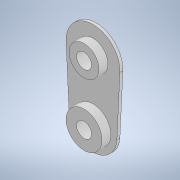
# Autodesk Inventor part: ヘッケン抑え
Saved by Autodesk Inventor 2022.2 (Build 262287030, 287C)
## iProperties
Created: 2022-01-09
Part Number: ヘッケン抑え
Material: Generic
Document SubType Name: Modeling
Designer: acps
Density: 1 g/cm^3
Appearance: Default
Author: acps
Autodesk Inventor part; units mm, degrees
ref_plane "YZ Plane" through (0, 0, 0) normal (1, 0, 0) x (0, 1, 0)
ref_plane "XZ Plane" through (0, 0, 0) normal (0, 1, 0) x (-1, 0, 0)
ref_plane "XY Plane" through (0, 0, 0) normal (0, 0, 1) x (1, 0, 0)
sketch "Sketch1" plane through (0, 0, 0) normal (0, 0, 1) x (1, 0, 0)
  circle A0 centre (0, 0) radius 2.5
  circle A1 centre (0, 0) radius 4.5
  circle A2 centre (0, -10) radius 1.25
  circle A3 centre (0, -10) radius 3
  circle A4 centre (0, -10) radius 4
  circle A5 centre (0, 0) radius 1.25
  line L0 (-4.4944, -0.225) -> (-3.995, -10.2)
  line L1 (4.4944, -0.225) -> (3.995, -10.2)
  line L2 (0, 0) -> (0, -19.0302) construction
  point P0 (66.1895, -52.0583)
  point P1 (148.6808, -39.1685)
  point P2 (99.1548, -7.9801)
  point P3 (101.772, -8.3287)
  point P4 (96.5376, -8.3287)
  dimension "d8" = 9
  dimension "d13" = 5
  dimension "d25" = 2.5
  dimension "d26" = 6
  dimension "d27" = 8
  dimension "d28" = 2.5
  dimension "d29" = 10
  constraints: 7 coincident, 6 centre point, 6 end point, 4 point on circle, 4 tangent, 1 point on line, 1 vertical
  measures "d8" diameter of A1
  measures "d13" diameter of A0
  measures "d25" diameter of A2
  measures "d26" diameter of A3
  measures "d27" diameter of A4
  measures "d28" diameter of A5
  measures "d29" distance of A2.centre point (0, 0)
extrude "Extrusion1" add sketch "Sketch1" along normal blind 0.5 contours A1 | A1 L1 A4 L0 | A4
extrude "Extrusion2" add sketch "Sketch1" along normal blind 2 contours A0 | A3
body "Solid1"
